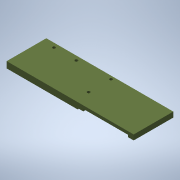
# Autodesk Inventor part: Oxxius laser subassy shortened baseplate
Saved by Autodesk Inventor 2022 (Build 260153000, 153)
## iProperties
Created: 2012-03-23
Part Number: Oxxius laser subassy shortened baseplate
Document SubType Name: Modeling
Designer: betzige
Density: 1 g/cm^3
Material: Generic
Appearance: Olive Drab
Author: betzige
Autodesk Inventor part; units mm, degrees
ref_plane "YZ Plane" through (0, 0, 0) normal (1, 0, 0) x (0, 1, 0)
ref_plane "XZ Plane" through (0, 0, 0) normal (0, 1, 0) x (-1, 0, 0)
ref_plane "XY Plane" through (0, 0, 0) normal (0, 0, 1) x (1, 0, 0)
sketch "Sketch1" plane through (0, 0, 0) normal (0, 0, 1) x (1, 0, 0)
  line L0 (-192.5, 35) -> (192.5, 35)
  line L1 (192.5, 35) -> (192.5, -55)
  line L2 (192.5, -55) -> (-192.5, -55)
  line L3 (-192.5, -55) -> (-192.5, 35)
  point P0 (0, 0)
  dimension "d0" = 385
  dimension "d1" = 192.5
  dimension "d2" = 90
  dimension "d3" = 55
  constraints: 8 end point, 2 parallel, 1 horizontal, 1 perpendicular
  measures "d0" distance of L0.start L0.end
  measures "d1" distance from line of point (0, 0) L3
  measures "d2" distance of L2.end L0.start
  measures "d3" distance from line of point (0, 0) L2
extrude "Extrusion1" add sketch "Sketch1" along normal blind 7
sketch "Sketch2" plane through (0, 0, 0) normal (0, 0, -1) x (-1, 0, 0)
  line L0 (192.5, 35) -> (-192.5, 35) projected
  line L1 (-192.5, 35) -> (-192.5, -55) projected
  line L2 (-192.5, -55) -> (192.5, -55) projected
  line L3 (17.417, 16.6256) -> (17.417, -16.6484) projected
  line L4 (-192.5, 16.6256) -> (-192.5, -16.6484) projected
  line L5 (17.417, 35) -> (17.417, -55)
  line L6 (4.717, 16.6256) -> (4.717, -16.6484) projected
  line L7 (-171.164, 18.034) -> (-179.8, 18.034) projected
  line L8 (-179.8, 16.6256) -> (-179.8, -16.6484) projected
  line L9 (-179.8, 35) -> (-179.8, -55)
  line L10 (4.717, 35) -> (4.717, -55)
  point P0 (0, 0)
  constraints: 6 end point, 6 point on line, 3 perpendicular
extrude "Extrusion2" add sketch "Sketch2" along normal blind 4.7408 contours L5 L3 L2 L10 L6 L0 | L9 L8 L2 L1 L0
sketch "Sketch3" plane through (0, 0, 0) normal (0, 0, -1) x (-1, 0, 0)
  line L0 (17.417, 35) -> (17.417, -55) projected
  line L1 (17.417, -55) -> (192.5, -55) projected
  line L2 (63.2414, 16.4628) -> (60.0979, -19.4679) projected
  line L3 (17.417, 35) -> (67.417, 35)
  line L4 (67.417, 35) -> (67.417, -55)
  line L5 (67.417, -55) -> (17.417, -55)
  line L6 (17.417, -55) -> (17.417, 35)
  line L7 (76.6696, -19.4) -> (76.6696, 30.6) projected
  line L8 (17.417, 35) -> (76.6696, 35)
  line L9 (76.6696, -55) -> (17.417, -55)
  line L10 (17.417, -55) -> (17.417, 35)
  circle A0 centre (83.6696, -4.5) radius 1.5 projected
  circle A1 centre (83.6696, 10.5) radius 2 projected
  line L11 (87.4689, -18.5) -> (87.4689, -24.5) projected
  line L12 (88.6696, -24.5) -> (87.4689, -24.5) projected
  line L13 (88.6696, 15.5) -> (88.6696, -24.5) projected
  line L14 (78.6696, 15.5) -> (88.6696, 15.5) projected
  line L15 (78.6696, -15.5) -> (78.6696, 15.5) projected
  line L16 (78.6696, -15.5) -> (84.4689, -15.5) projected
  arc A2 (87.4689, -18.5) -> (84.4689, -15.5) centre (84.4689, -18.5) ccw projected
  line L17 (67.417, 35) -> (78.6696, 35)
  line L18 (78.6696, 35) -> (78.6696, -55)
  line L19 (78.6696, -55) -> (67.417, -55)
  line L20 (67.417, -55) -> (67.417, 35)
  point P0 (0, 0)
  dimension "d8" = 50
  dimension "d11" = 0
  constraints: 22 end point, 5 parallel, 3 horizontal, 2 perpendicular, 2 point on line
  measures "d8" distance between parallel lines of L6 L4
  measures "d11" distance between parallel lines of L1 L9
extrude "Extrusion3" add sketch "Sketch3" along normal blind 7.3198 contours L3 L4 L1 L0 | L8 L17 L18 L15 L1 L4
sketch "Sketch6" plane through (-192.5, -55, 7) normal (-1, 0, 0) x (0, 0, 1)
  line L0 (-23, 0) -> (-23, 65) projected
  circle A0 centre (-28, 23.1) radius 1.2295 projected
  circle A1 centre (-28, 53.1) radius 1.2295 projected
  point P0 (-7, 55)
  constraints: 2 coincident
hole "Hole1" at (-192.5, -31.9, -21) at (-192.5, -1.9, -21) direction (1, 0, 0) diameter 3 end through all counterbore diameter 5.75 counterbore depth 3
sketch "Sketch8" plane through (0, 0, 7) normal (0, 0, 1) x (1, 0, 0)
  circle A0 centre (-57.2416, -1.1152) radius 2.0828 projected
  circle A1 centre (-33.7068, 0.9439) radius 2.0828 projected
  point P0 (0, 0)
  constraints: 2 coincident
hole "Hole3" [suppressed]
sketch "Sketch9" plane through (0, 0, -4.7408) normal (0, 0, -1) x (-1, 0, 0)
  circle A0 centre (11.067, -7.6314) radius 2.1844 projected
  circle A1 centre (11.067, 7.6086) radius 2.1844 projected
  circle A2 centre (-186.15, -7.6314) radius 2.1844 projected
  circle A3 centre (-186.15, 7.6086) radius 2.1844 projected
  point P0 (0, 0)
  constraints: 4 coincident
hole "Hole4" at (-11.067, -7.6314, -4.7408) at (-11.067, 7.6086, -4.7408) at (186.15, -7.6314, -4.7408) at (186.15, 7.6086, -4.7408) direction (0, 0, 1) diameter 3.302 depth 8 tip angle 118 thread size "8-32 UNC" class "2B" standard "ANSI Unified Screw Threads"
sketch "Sketch10" plane through (0, 0, 0) normal (0, 0, -1) x (-1, 0, 0)
  line L0 (192.5, 35) -> (78.6696, 35) projected
  line L1 (178.6696, 15.5) -> (178.6696, -24.5) projected
  line L2 (178.6696, 35) -> (192.5, 35)
  line L3 (192.5, 35) -> (192.5, -55)
  line L4 (192.5, -55) -> (178.6696, -55)
  line L5 (178.6696, -55) -> (178.6696, 35)
  point P0 (0, 0)
  constraints: 8 end point, 2 parallel, 1 horizontal, 1 perpendicular, 1 point on line
extrude "Extrusion6" cut sketch "Sketch10" against normal blind 10
sketch "Sketch11" plane through (0, 0, 0) normal (0, 0, -1) x (-1, 0, 0)
  line L0 (178.6696, -55) -> (178.6696, 35) projected
  line L1 (178.6696, 35) -> (78.6696, 35) projected
  line L2 (78.6696, 35) -> (78.6696, -55) projected
  line L3 (78.6696, -55) -> (178.6696, -55) projected
  point P0 (0, 0)
extrude "Extrusion7" add sketch "Sketch11" along normal blind 7.3198
sketch "Sketch12" plane through (0, 0, -7.3198) normal (0, 0, -1) x (-1, 0, 0)
  circle A0 centre (173.6696, 10.5) radius 2 projected
  line L0 (78.6696, 15.5) -> (178.6696, 15.5) projected
  line L1 (178.6696, 15.5) -> (178.6696, -24.5) projected
  line L2 (178.6696, -24.5) -> (78.6696, -24.5) projected
  line L3 (78.6696, -24.5) -> (78.6696, 15.5) projected
  circle A1 centre (173.6696, -44.5) radius 2.0242
  circle A2 centre (58.6696, 10.5) radius 2.0032
  circle A3 centre (58.6696, -44.5) radius 2.0032
  point P0 (0, 0)
  dimension "d126" = 55
  dimension "d127" = 115
  constraints: 3 centre point, 1 coincident
  measures "d126" distance of A1.centre A0.centre
  measures "d127" distance of A2.centre A0.centre
hole "Hole5" at (-173.6696, 10.5, -7.3198) direction (0, 0, 1) diameter 2.459 depth 8.8 tip angle 118 thread size "M3x0.5" class "6H" standard "ANSI Metric M Profile"
sketch "Sketch13" plane through (0, 0, -7.3198) normal (0, 0, -1) x (-1, 0, 0)
  line L0 (171.6696, -6) -> (175.6696, -6) projected
  arc A0 (175.6696, -6) -> (175.6696, -3) centre (175.6696, -4.5) ccw projected
  line L1 (175.6696, -3) -> (171.6696, -3) projected
  arc A1 (171.6696, -3) -> (171.6696, -6) centre (171.6696, -4.5) ccw projected
  circle A2 centre (83.6696, -4.5) radius 1.5 projected
  circle A3 centre (173.6696, 10.5) radius 2 projected
  circle A4 centre (173.6696, -19.5) radius 2 projected
  circle A5 centre (83.6696, 10.5) radius 2 projected
  circle A6 centre (83.6696, -19.5) radius 2 projected
  line L2 (78.6696, 15.5) -> (178.6696, 15.5) projected
  line L3 (178.6696, 15.5) -> (178.6696, -24.5) projected
  line L4 (178.6696, -24.5) -> (78.6696, -24.5) projected
  line L5 (78.6696, -24.5) -> (78.6696, 15.5) projected
  point P0 (0, 0)
  point P1 (173.6696, -4.5)
  constraints: 1 coincident
hole "Hole6" [suppressed]
sketch "Sketch14" plane through (0, 0, -7.3198) normal (0, 0, -1) x (-1, 0, 0)
  circle A0 centre (126.3, 25.4) radius 3.175 projected
  circle A1 centre (151.7, 25.4) radius 3.175 projected
  point P0 (0, 0)
  point P1 (100.9, 25.4)
  dimension "d63" = 50.8
  constraints: 1 coincident
  measures "d63" distance of point (151.7, 25.4) point (100.9, 25.4)
hole "Hole7" at (-151.7, 25.4, -7.3198) at (-100.9, 25.4, -7.3198) direction (0, 0, 1) diameter 6.35 end through all counterbore diameter 9.652 counterbore depth 7
sketch "Sketch15" plane through (0, 0, -7.3198) normal (0, 0, -1) x (-1, 0, 0)
  line L0 (17.417, 35) -> (78.6696, 35) projected
  circle A0 centre (100.9, 25.4) radius 4.826 projected
  point P0 (0, 0)
  point P1 (24.741, 27.9)
  point P2 (24.7, -22.9)
  dimension "d71" = 7.1
  dimension "d72" = 76.2
  dimension "d73" = 76.2
  dimension "d74" = 50.8
  measures "d71" distance from line of L0 point (24.741, 27.9)
  measures "d72" distance of A0.centre point (24.741, 27.9)
  measures "d73" horizontal distance of A0.centre point (24.7, -22.9)
  measures "d74" distance of point (24.741, 27.9) point (24.7, -22.9)
hole "Hole8" at (-24.741, 27.9, -7.3198) at (-24.7, -22.9, -7.3198) direction (0, 0, 1) diameter 6.35 end through all counterbore diameter 9.652 counterbore depth 7
sketch "Sketch17" plane through (0, 0, 0) normal (0, 0, -1) x (-1, 0, 0)
  line L0 (-179.8, -55) -> (4.717, -55) projected
  line L1 (4.717, 35) -> (-179.8, 35) projected
  line L2 (-109.583, 16.6256) -> (-109.583, -16.6484) projected
  line L3 (-96.883, 16.6256) -> (-96.883, -16.6484) projected
  line L4 (-96.883, 35) -> (-109.583, 35)
  line L5 (-109.583, 35) -> (-109.583, -55)
  line L6 (-109.583, -55) -> (-96.883, -55)
  line L7 (-96.883, -55) -> (-96.883, 35)
  point P0 (0, 0)
  constraints: 8 end point, 2 parallel, 2 point on line, 1 horizontal, 1 perpendicular
extrude "Extrusion8" add sketch "Sketch17" along normal blind 4.7408
sketch "Sketch18" plane through (0, 0, -4.7408) normal (0, 0, -1) x (-1, 0, 0)
  circle A0 centre (-103.233, -7.6314) radius 2.1844 projected
  circle A1 centre (-103.233, 7.6086) radius 2.1844 projected
  point P0 (0, 0)
hole "Hole10" at (103.233, -7.6314, -4.7408) at (103.233, 7.6086, -4.7408) direction (0, 0, 1) diameter 3.302 depth 8 tip angle 118 thread size "8-32 UNC" class "2B" standard "ANSI Unified Screw Threads"
sketch "Sketch19" plane through (0, 0, -4.7408) normal (0, 0, -1) x (-1, 0, 0)
  line L0 (-192.5, -55) -> (-192.5, 35) projected
  line L1 (-179.8, -55) -> (-109.583, -55) projected
  line L2 (-109.583, 35) -> (-179.8, 35) projected
  line L3 (-109.583, 35) -> (-192.5, 35)
  line L4 (-192.5, 35) -> (-192.5, -55)
  line L5 (-192.5, -55) -> (-109.583, -55)
  line L6 (-109.583, -55) -> (-109.583, 35)
  point P0 (0, 0)
  constraints: 8 end point, 2 parallel, 1 horizontal, 1 perpendicular
extrude "Extrusion9" cut sketch "Sketch19" against normal blind 25
sketch "Sketch20" plane through (0, 0, 0) normal (0, 0, -1) x (-1, 0, 0)
  circle A0 centre (24.7, -22.9) radius 4.826 projected
  circle A1 centre (24.741, 27.9) radius 4.826 projected
  point P0 (0, 0)
  point P1 (-76.9, -22.9)
  point P2 (-76.859, 27.9)
  dimension "d103" = 101.6
  dimension "d104" = 101.6
  measures "d103" distance of A0.centre point (-76.9, -22.9)
  measures "d104" distance of A1.centre point (-76.859, 27.9)
hole "Hole11" [suppressed]
hole "Hole12" [suppressed]
hole "Hole13" [suppressed]
hole "Hole14" at (-173.6696, -44.5, -7.3198) direction (0, 0, 1) diameter 2.459 depth 8.8 tip angle 118 thread size "M3x0.5" class "6H" standard "ANSI Metric M Profile"
hole "Hole15" at (-58.6696, 10.5, -7.3198) direction (0, 0, 1) diameter 2.459 depth 8.8 tip angle 118 thread size "M3x0.5" class "6H" standard "ANSI Metric M Profile"
hole "Hole16" at (-58.6696, -44.5, -7.3198) direction (0, 0, 1) diameter 2.459 depth 8.8 tip angle 118 thread size "M3x0.5" class "6H" standard "ANSI Metric M Profile"
body "Solid1"
